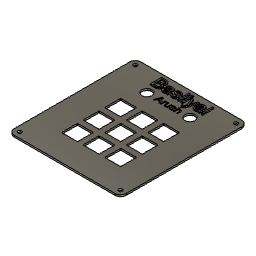
top part (Autodesk Fusion 360 design; units mm, degrees)
Autodesk Fusion 360 part; units mm, degrees
note: some values were not read from the file. Set by a fixed rule: which sketch regions a step uses.
(part 1 of 2)
sketch "plate-2025-07-12T03_53_15.257Z" plane through (0, 0, 0) normal (0, 0, 1) x (1, 0, 0)
  line L0 (3.025, -21.575) -> (16.025, -21.575)
  line L1 (3.025, -35.575) -> (16.025, -35.575)
  line L2 (2.525, -22.075) -> (2.525, -35.075)
  line L3 (16.525, -22.075) -> (16.525, -35.075)
  arc A0 (3.025, -21.575) -> (2.525, -22.075) centre (3.025, -22.075) ccw
  arc A1 (16.525, -22.075) -> (16.025, -21.575) centre (16.025, -22.075) ccw
  arc A2 (2.525, -35.075) -> (3.025, -35.575) centre (3.025, -35.075) ccw
  arc A3 (16.025, -35.575) -> (16.525, -35.075) centre (16.025, -35.075) ccw
  line L4 (22.075, -21.575) -> (35.075, -21.575)
  line L5 (22.075, -35.575) -> (35.075, -35.575)
  line L6 (21.575, -22.075) -> (21.575, -35.075)
  line L7 (35.575, -22.075) -> (35.575, -35.075)
  arc A4 (22.075, -21.575) -> (21.575, -22.075) centre (22.075, -22.075) ccw
  arc A5 (35.575, -22.075) -> (35.075, -21.575) centre (35.075, -22.075) ccw
  arc A6 (21.575, -35.075) -> (22.075, -35.575) centre (22.075, -35.075) ccw
  arc A7 (35.075, -35.575) -> (35.575, -35.075) centre (35.075, -35.075) ccw
  line L8 (41.125, -21.575) -> (54.125, -21.575)
  line L9 (41.125, -35.575) -> (54.125, -35.575)
  line L10 (40.625, -22.075) -> (40.625, -35.075)
  line L11 (54.625, -22.075) -> (54.625, -35.075)
  arc A8 (41.125, -21.575) -> (40.625, -22.075) centre (41.125, -22.075) ccw
  arc A9 (54.625, -22.075) -> (54.125, -21.575) centre (54.125, -22.075) ccw
  arc A10 (40.625, -35.075) -> (41.125, -35.575) centre (41.125, -35.075) ccw
  arc A11 (54.125, -35.575) -> (54.625, -35.075) centre (54.125, -35.075) ccw
  line L12 (3.025, -40.625) -> (16.025, -40.625)
  line L13 (3.025, -54.625) -> (16.025, -54.625)
  line L14 (2.525, -41.125) -> (2.525, -54.125)
  line L15 (16.525, -41.125) -> (16.525, -54.125)
  arc A12 (3.025, -40.625) -> (2.525, -41.125) centre (3.025, -41.125) ccw
  arc A13 (16.525, -41.125) -> (16.025, -40.625) centre (16.025, -41.125) ccw
  arc A14 (2.525, -54.125) -> (3.025, -54.625) centre (3.025, -54.125) ccw
  arc A15 (16.025, -54.625) -> (16.525, -54.125) centre (16.025, -54.125) ccw
  line L16 (22.075, -40.625) -> (35.075, -40.625)
  line L17 (22.075, -54.625) -> (35.075, -54.625)
  line L18 (21.575, -41.125) -> (21.575, -54.125)
  line L19 (35.575, -41.125) -> (35.575, -54.125)
  arc A16 (22.075, -40.625) -> (21.575, -41.125) centre (22.075, -41.125) ccw
  arc A17 (35.575, -41.125) -> (35.075, -40.625) centre (35.075, -41.125) ccw
  arc A18 (21.575, -54.125) -> (22.075, -54.625) centre (22.075, -54.125) ccw
  arc A19 (35.075, -54.625) -> (35.575, -54.125) centre (35.075, -54.125) ccw
  line L20 (41.125, -40.625) -> (54.125, -40.625)
  line L21 (41.125, -54.625) -> (54.125, -54.625)
  line L22 (40.625, -41.125) -> (40.625, -54.125)
  line L23 (54.625, -41.125) -> (54.625, -54.125)
  arc A20 (41.125, -40.625) -> (40.625, -41.125) centre (41.125, -41.125) ccw
  arc A21 (54.625, -41.125) -> (54.125, -40.625) centre (54.125, -41.125) ccw
  arc A22 (40.625, -54.125) -> (41.125, -54.625) centre (41.125, -54.125) ccw
  arc A23 (54.125, -54.625) -> (54.625, -54.125) centre (54.125, -54.125) ccw
  line L24 (3.025, -59.675) -> (16.025, -59.675)
  line L25 (3.025, -73.675) -> (16.025, -73.675)
  line L26 (2.525, -60.175) -> (2.525, -73.175)
  line L27 (16.525, -60.175) -> (16.525, -73.175)
  arc A24 (3.025, -59.675) -> (2.525, -60.175) centre (3.025, -60.175) ccw
  arc A25 (16.525, -60.175) -> (16.025, -59.675) centre (16.025, -60.175) ccw
  arc A26 (2.525, -73.175) -> (3.025, -73.675) centre (3.025, -73.175) ccw
  arc A27 (16.025, -73.675) -> (16.525, -73.175) centre (16.025, -73.175) ccw
  line L28 (22.075, -59.675) -> (35.075, -59.675)
  line L29 (22.075, -73.675) -> (35.075, -73.675)
  line L30 (21.575, -60.175) -> (21.575, -73.175)
  line L31 (35.575, -60.175) -> (35.575, -73.175)
  arc A28 (22.075, -59.675) -> (21.575, -60.175) centre (22.075, -60.175) ccw
  arc A29 (35.575, -60.175) -> (35.075, -59.675) centre (35.075, -60.175) ccw
  arc A30 (21.575, -73.175) -> (22.075, -73.675) centre (22.075, -73.175) ccw
  arc A31 (35.075, -73.675) -> (35.575, -73.175) centre (35.075, -73.175) ccw
  line L32 (41.125, -59.675) -> (54.125, -59.675)
  line L33 (41.125, -73.675) -> (54.125, -73.675)
  line L34 (40.625, -60.175) -> (40.625, -73.175)
  line L35 (54.625, -60.175) -> (54.625, -73.175)
  arc A32 (41.125, -59.675) -> (40.625, -60.175) centre (41.125, -60.175) ccw
  arc A33 (54.625, -60.175) -> (54.125, -59.675) centre (54.125, -60.175) ccw
  arc A34 (40.625, -73.175) -> (41.125, -73.675) centre (41.125, -73.175) ccw
  arc A35 (54.125, -73.675) -> (54.625, -73.175) centre (54.125, -73.175) ccw
sketch "Sketch2" plane through (0, 0, 0) normal (0, 0, 1) x (1, 0, 0)
  line L0 (-21.36, 15.31) -> (77.64, 15.31)
  line L1 (77.64, 15.31) -> (77.64, -96.69)
  line L2 (77.64, -96.69) -> (-21.36, -96.69)
  line L3 (-21.36, -96.69) -> (-21.36, 15.31)
  line L4 (54.625, -60.175) -> (54.625, -73.175)
  line L5 (41.125, -73.675) -> (54.125, -73.675)
  dimension "d1" = 99
  dimension "d2" = 112
  dimension "d3" = 23.015
  dimension "d4" = 23.015
  constraint horizontal L0
  constraint vertical L1
  constraint horizontal L2
  constraint vertical L3
  measures "d1" distance of L0.start L0.end
  measures "d2" distance of L0.start L2.end
  measures "d3" distance of L1 L4
  measures "d4" distance of L2 L5
sketch "Sketch3" plane through (0, 0, 0) normal (0, 0, 1) x (1, 0, 0)
  circle A0 centre (-16.36, 10.31) radius 1.7
  line L0 (-21.36, 15.31) -> (77.64, 15.31)
  line L1 (-21.36, -96.69) -> (-21.36, 15.31)
  circle A1 centre (72.64, 10.31) radius 1.7
  circle A2 centre (-16.36, -91.69) radius 1.7
  circle A3 centre (72.64, -91.69) radius 1.7
  dimension "d6" = 3.4
  dimension "d7" = 5
  dimension "d8" = 5
  measures "d6" diameter of A0
  measures "d7" distance of A0.centre L0
  measures "d8" distance of A0.centre L1
extrude "Extrude1" add sketch "Sketch2" along normal blind 1.5
extrude "Extrude2" cut sketch "plate-2025-07-12T03_53_15.257Z" sketch "Sketch3" along normal blind 1.5 of sketch 2
sketch "Sketch4" plane through (0, 0, 1.5) normal (0, 0, 1) x (-1, 0, 0)
  circle A0 centre (-72.64, 91.69) radius 1.7
  circle A1 centre (16.36, -10.31) radius 1.7
  line L0 (-41.125, 59.675) -> (-54.125, 59.675)
  arc A2 (-54.625, 60.175) -> (-54.125, 59.675) centre (-54.125, 60.175) ccw
  line L1 (-54.625, 60.175) -> (-54.625, 73.175)
  arc A3 (-54.125, 73.675) -> (-54.625, 73.175) centre (-54.125, 73.175) ccw
  line L2 (-54.125, 73.675) -> (-41.125, 73.675)
  arc A4 (-40.625, 73.175) -> (-41.125, 73.675) centre (-41.125, 73.175) ccw
  line L3 (-40.625, 73.175) -> (-40.625, 60.175)
  arc A5 (-41.125, 59.675) -> (-40.625, 60.175) centre (-41.125, 60.175) ccw
  line L4 (-3.025, 21.575) -> (-16.025, 21.575)
  arc A6 (-16.525, 22.075) -> (-16.025, 21.575) centre (-16.025, 22.075) ccw
  line L5 (-16.525, 22.075) -> (-16.525, 35.075)
  arc A7 (-16.025, 35.575) -> (-16.525, 35.075) centre (-16.025, 35.075) ccw
  line L6 (-16.025, 35.575) -> (-3.025, 35.575)
  arc A8 (-2.525, 35.075) -> (-3.025, 35.575) centre (-3.025, 35.075) ccw
  line L7 (-2.525, 35.075) -> (-2.525, 22.075)
  arc A9 (-3.025, 21.575) -> (-2.525, 22.075) centre (-3.025, 22.075) ccw
  line L8 (-22.075, 21.575) -> (-35.075, 21.575)
  arc A10 (-35.575, 22.075) -> (-35.075, 21.575) centre (-35.075, 22.075) ccw
  line L9 (-35.575, 22.075) -> (-35.575, 35.075)
  arc A11 (-35.075, 35.575) -> (-35.575, 35.075) centre (-35.075, 35.075) ccw
  line L10 (-35.075, 35.575) -> (-22.075, 35.575)
  arc A12 (-21.575, 35.075) -> (-22.075, 35.575) centre (-22.075, 35.075) ccw
  line L11 (-21.575, 35.075) -> (-21.575, 22.075)
  arc A13 (-22.075, 21.575) -> (-21.575, 22.075) centre (-22.075, 22.075) ccw
  line L12 (-41.125, 40.625) -> (-54.125, 40.625)
  arc A14 (-54.625, 41.125) -> (-54.125, 40.625) centre (-54.125, 41.125) ccw
  line L13 (-54.625, 41.125) -> (-54.625, 54.125)
  arc A15 (-54.125, 54.625) -> (-54.625, 54.125) centre (-54.125, 54.125) ccw
  line L14 (-54.125, 54.625) -> (-41.125, 54.625)
  arc A16 (-40.625, 54.125) -> (-41.125, 54.625) centre (-41.125, 54.125) ccw
  line L15 (-40.625, 54.125) -> (-40.625, 41.125)
  arc A17 (-41.125, 40.625) -> (-40.625, 41.125) centre (-41.125, 41.125) ccw
  line L16 (-22.075, 59.675) -> (-35.075, 59.675)
  arc A18 (-35.575, 60.175) -> (-35.075, 59.675) centre (-35.075, 60.175) ccw
  line L17 (-35.575, 60.175) -> (-35.575, 73.175)
  arc A19 (-35.075, 73.675) -> (-35.575, 73.175) centre (-35.075, 73.175) ccw
  line L18 (-35.075, 73.675) -> (-22.075, 73.675)
  arc A20 (-21.575, 73.175) -> (-22.075, 73.675) centre (-22.075, 73.175) ccw
  line L19 (-21.575, 73.175) -> (-21.575, 60.175)
  arc A21 (-22.075, 59.675) -> (-21.575, 60.175) centre (-22.075, 60.175) ccw
  line L20 (-3.025, 40.625) -> (-16.025, 40.625)
  arc A22 (-16.525, 41.125) -> (-16.025, 40.625) centre (-16.025, 41.125) ccw
  line L21 (-16.525, 41.125) -> (-16.525, 54.125)
  arc A23 (-16.025, 54.625) -> (-16.525, 54.125) centre (-16.025, 54.125) ccw
  line L22 (-16.025, 54.625) -> (-3.025, 54.625)
  arc A24 (-2.525, 54.125) -> (-3.025, 54.625) centre (-3.025, 54.125) ccw
  line L23 (-2.525, 54.125) -> (-2.525, 41.125)
  arc A25 (-3.025, 40.625) -> (-2.525, 41.125) centre (-3.025, 41.125) ccw
  line L24 (-41.125, 21.575) -> (-54.125, 21.575)
  arc A26 (-54.625, 22.075) -> (-54.125, 21.575) centre (-54.125, 22.075) ccw
  line L25 (-54.625, 22.075) -> (-54.625, 35.075)
  arc A27 (-54.125, 35.575) -> (-54.625, 35.075) centre (-54.125, 35.075) ccw
  line L26 (-54.125, 35.575) -> (-41.125, 35.575)
  arc A28 (-40.625, 35.075) -> (-41.125, 35.575) centre (-41.125, 35.075) ccw
  line L27 (-40.625, 35.075) -> (-40.625, 22.075)
  arc A29 (-41.125, 21.575) -> (-40.625, 22.075) centre (-41.125, 22.075) ccw
  line L28 (-22.075, 40.625) -> (-35.075, 40.625)
  arc A30 (-35.575, 41.125) -> (-35.075, 40.625) centre (-35.075, 41.125) ccw
  line L29 (-35.575, 41.125) -> (-35.575, 54.125)
  arc A31 (-35.075, 54.625) -> (-35.575, 54.125) centre (-35.075, 54.125) ccw
  line L30 (-35.075, 54.625) -> (-22.075, 54.625)
  arc A32 (-21.575, 54.125) -> (-22.075, 54.625) centre (-22.075, 54.125) ccw
  line L31 (-21.575, 54.125) -> (-21.575, 41.125)
  arc A33 (-22.075, 40.625) -> (-21.575, 41.125) centre (-22.075, 41.125) ccw
  line L32 (-3.025, 59.675) -> (-16.025, 59.675)
  arc A34 (-16.525, 60.175) -> (-16.025, 59.675) centre (-16.025, 60.175) ccw
  line L33 (-16.525, 60.175) -> (-16.525, 73.175)
  arc A35 (-16.025, 73.675) -> (-16.525, 73.175) centre (-16.025, 73.175) ccw
  line L34 (-16.025, 73.675) -> (-3.025, 73.675)
  arc A36 (-2.525, 73.175) -> (-3.025, 73.675) centre (-3.025, 73.175) ccw
  line L35 (-2.525, 73.175) -> (-2.525, 60.175)
  arc A37 (-3.025, 59.675) -> (-2.525, 60.175) centre (-3.025, 60.175) ccw
  circle A38 centre (16.36, 91.69) radius 1.7
  circle A39 centre (-72.64, -10.31) radius 1.7
  line L36 (21.36, 96.69) -> (-77.64, 96.69)
  line L37 (-77.64, 96.69) -> (-77.64, -15.31)
  line L38 (-77.64, -15.31) -> (21.36, -15.31)
  line L39 (21.36, -15.31) -> (21.36, 96.69)
  line L40 (-28.14, -15.31) -> (-28.14, 96.69)
  line L41 (-47.625, 28.575) -> (-28.14, 28.575)
  line L42 (-35.575, 47.625) -> (-28.14, 47.625)
  line L43 (-28.14, 47.625) -> (-28.14, 28.575)
  line L44 (-28.14, 28.575) -> (-28.14, 9.525)
  line L45 (-28.14, 9.525) -> (-47.625, 9.525)
  circle A40 centre (-47.625, 9.525) radius 4.25
  circle A41 centre (-8.655, 9.525) radius 4.25
  dimension "d13" = 19.05
  dimension "d14" = 8.5
  constraint midpoint L38 L40.start
  constraint midpoint L36 L40.end
  constraint coincident L40 L41.end
  constraint perpendicular L40 L41
  constraint midpoint L29 L42.start
  constraint coincident L40 L42.end
  constraint perpendicular L40 L42
  constraint perpendicular L41 L44
  constraint perpendicular L44 L45
  constraint coincident L45.end A40.centre
  constraint symmetric L40 A40 A41
  measures "d13" distance of L41.end L44.end
  measures "d14" diameter of A40
extrude "Extrude3" cut sketch "Sketch4" against normal blind 12 contours A40 | A41
fillet "Fillet1" radius 5 4 edges at (-21.36, -96.69, 0.75) (77.64, -96.69, 0.75) (77.64, 15.31, 0.75) (-21.36, 15.31, 0.75)
sketch "Sketch8" plane through (0, 0, 1.5) normal (0, 0, 1) x (-1, 0, 0)
  arc A0 (16.36, -15.31) -> (21.36, -10.31) centre (16.36, -10.31) ccw
  line L0 (21.36, -10.31) -> (21.36, 91.69)
  arc A1 (21.36, 91.69) -> (16.36, 96.69) centre (16.36, 91.69) ccw
  line L1 (16.36, 96.69) -> (-72.64, 96.69)
  arc A2 (-72.64, 96.69) -> (-77.64, 91.69) centre (-72.64, 91.69) ccw
  line L2 (-77.64, 91.69) -> (-77.64, -10.31)
  arc A3 (-77.64, -10.31) -> (-72.64, -15.31) centre (-72.64, -10.31) ccw
  line L3 (-72.64, -15.31) -> (16.36, -15.31)
  circle A4 centre (-72.64, -10.31) radius 1.7
  circle A5 centre (16.36, 91.69) radius 1.7
  line L4 (-3.025, 59.675) -> (-16.025, 59.675)
  arc A6 (-16.525, 60.175) -> (-16.025, 59.675) centre (-16.025, 60.175) ccw
  line L5 (-16.525, 60.175) -> (-16.525, 73.175)
  arc A7 (-16.025, 73.675) -> (-16.525, 73.175) centre (-16.025, 73.175) ccw
  line L6 (-16.025, 73.675) -> (-3.025, 73.675)
  arc A8 (-2.525, 73.175) -> (-3.025, 73.675) centre (-3.025, 73.175) ccw
  line L7 (-2.525, 73.175) -> (-2.525, 60.175)
  arc A9 (-3.025, 59.675) -> (-2.525, 60.175) centre (-3.025, 60.175) ccw
  line L8 (-22.075, 40.625) -> (-35.075, 40.625)
  arc A10 (-35.575, 41.125) -> (-35.075, 40.625) centre (-35.075, 41.125) ccw
  line L9 (-35.575, 41.125) -> (-35.575, 54.125)
  arc A11 (-35.075, 54.625) -> (-35.575, 54.125) centre (-35.075, 54.125) ccw
  line L10 (-35.075, 54.625) -> (-22.075, 54.625)
  arc A12 (-21.575, 54.125) -> (-22.075, 54.625) centre (-22.075, 54.125) ccw
  line L11 (-21.575, 54.125) -> (-21.575, 41.125)
  arc A13 (-22.075, 40.625) -> (-21.575, 41.125) centre (-22.075, 41.125) ccw
  line L12 (-41.125, 21.575) -> (-54.125, 21.575)
  arc A14 (-54.625, 22.075) -> (-54.125, 21.575) centre (-54.125, 22.075) ccw
  line L13 (-54.625, 22.075) -> (-54.625, 35.075)
  arc A15 (-54.125, 35.575) -> (-54.625, 35.075) centre (-54.125, 35.075) ccw
  line L14 (-54.125, 35.575) -> (-41.125, 35.575)
  arc A16 (-40.625, 35.075) -> (-41.125, 35.575) centre (-41.125, 35.075) ccw
  line L15 (-40.625, 35.075) -> (-40.625, 22.075)
  arc A17 (-41.125, 21.575) -> (-40.625, 22.075) centre (-41.125, 22.075) ccw
  line L16 (-3.025, 40.625) -> (-16.025, 40.625)
  arc A18 (-16.525, 41.125) -> (-16.025, 40.625) centre (-16.025, 41.125) ccw
  line L17 (-16.525, 41.125) -> (-16.525, 54.125)
  arc A19 (-16.025, 54.625) -> (-16.525, 54.125) centre (-16.025, 54.125) ccw
  line L18 (-16.025, 54.625) -> (-3.025, 54.625)
  arc A20 (-2.525, 54.125) -> (-3.025, 54.625) centre (-3.025, 54.125) ccw
  line L19 (-2.525, 54.125) -> (-2.525, 41.125)
  arc A21 (-3.025, 40.625) -> (-2.525, 41.125) centre (-3.025, 41.125) ccw
  line L20 (-22.075, 59.675) -> (-35.075, 59.675)
  arc A22 (-35.575, 60.175) -> (-35.075, 59.675) centre (-35.075, 60.175) ccw
  line L21 (-35.575, 60.175) -> (-35.575, 73.175)
  arc A23 (-35.075, 73.675) -> (-35.575, 73.175) centre (-35.075, 73.175) ccw
  line L22 (-35.075, 73.675) -> (-22.075, 73.675)
  arc A24 (-21.575, 73.175) -> (-22.075, 73.675) centre (-22.075, 73.175) ccw
  line L23 (-21.575, 73.175) -> (-21.575, 60.175)
  arc A25 (-22.075, 59.675) -> (-21.575, 60.175) centre (-22.075, 60.175) ccw
  line L24 (-41.125, 40.625) -> (-54.125, 40.625)
  arc A26 (-54.625, 41.125) -> (-54.125, 40.625) centre (-54.125, 41.125) ccw
  line L25 (-54.625, 41.125) -> (-54.625, 54.125)
  arc A27 (-54.125, 54.625) -> (-54.625, 54.125) centre (-54.125, 54.125) ccw
  line L26 (-54.125, 54.625) -> (-41.125, 54.625)
  arc A28 (-40.625, 54.125) -> (-41.125, 54.625) centre (-41.125, 54.125) ccw
  line L27 (-40.625, 54.125) -> (-40.625, 41.125)
  arc A29 (-41.125, 40.625) -> (-40.625, 41.125) centre (-41.125, 41.125) ccw
  line L28 (-22.075, 21.575) -> (-35.075, 21.575)
  arc A30 (-35.575, 22.075) -> (-35.075, 21.575) centre (-35.075, 22.075) ccw
  line L29 (-35.575, 22.075) -> (-35.575, 35.075)
  arc A31 (-35.075, 35.575) -> (-35.575, 35.075) centre (-35.075, 35.075) ccw
  line L30 (-35.075, 35.575) -> (-22.075, 35.575)
  arc A32 (-21.575, 35.075) -> (-22.075, 35.575) centre (-22.075, 35.075) ccw
  line L31 (-21.575, 35.075) -> (-21.575, 22.075)
  arc A33 (-22.075, 21.575) -> (-21.575, 22.075) centre (-22.075, 22.075) ccw
  line L32 (-3.025, 21.575) -> (-16.025, 21.575)
  arc A34 (-16.525, 22.075) -> (-16.025, 21.575) centre (-16.025, 22.075) ccw
  line L33 (-16.525, 22.075) -> (-16.525, 35.075)
  arc A35 (-16.025, 35.575) -> (-16.525, 35.075) centre (-16.025, 35.075) ccw
  line L34 (-16.025, 35.575) -> (-3.025, 35.575)
  arc A36 (-2.525, 35.075) -> (-3.025, 35.575) centre (-3.025, 35.075) ccw
  line L35 (-2.525, 35.075) -> (-2.525, 22.075)
  arc A37 (-3.025, 21.575) -> (-2.525, 22.075) centre (-3.025, 22.075) ccw
  line L36 (-41.125, 59.675) -> (-54.125, 59.675)
  arc A38 (-54.625, 60.175) -> (-54.125, 59.675) centre (-54.125, 60.175) ccw
  line L37 (-54.625, 60.175) -> (-54.625, 73.175)
  arc A39 (-54.125, 73.675) -> (-54.625, 73.175) centre (-54.125, 73.175) ccw
  line L38 (-54.125, 73.675) -> (-41.125, 73.675)
  arc A40 (-40.625, 73.175) -> (-41.125, 73.675) centre (-41.125, 73.175) ccw
  line L39 (-40.625, 73.175) -> (-40.625, 60.175)
  arc A41 (-41.125, 59.675) -> (-40.625, 60.175) centre (-41.125, 60.175) ccw
  circle A42 centre (16.36, -10.31) radius 1.7
  circle A43 centre (-72.64, 91.69) radius 1.7
  circle A44 centre (-8.655, 9.525) radius 4.25
  circle A45 centre (-47.625, 9.525) radius 4.25
sketch "Sketch9" plane through (0, 0, 1.5) normal (0, 0, 1) x (-1, 0, 0)
  arc A0 (16.36, -15.31) -> (21.36, -10.31) centre (16.36, -10.31) ccw
  line L0 (21.36, -10.31) -> (21.36, 91.69)
  arc A1 (21.36, 91.69) -> (16.36, 96.69) centre (16.36, 91.69) ccw
  line L1 (16.36, 96.69) -> (-72.64, 96.69)
  arc A2 (-72.64, 96.69) -> (-77.64, 91.69) centre (-72.64, 91.69) ccw
  line L2 (-77.64, 91.69) -> (-77.64, -10.31)
  arc A3 (-77.64, -10.31) -> (-72.64, -15.31) centre (-72.64, -10.31) ccw
  line L3 (-72.64, -15.31) -> (16.36, -15.31)
  circle A4 centre (-72.64, -10.31) radius 1.7
  circle A5 centre (16.36, 91.69) radius 1.7
  line L4 (-3.025, 59.675) -> (-16.025, 59.675)
  arc A6 (-16.525, 60.175) -> (-16.025, 59.675) centre (-16.025, 60.175) ccw
  line L5 (-16.525, 60.175) -> (-16.525, 73.175)
  arc A7 (-16.025, 73.675) -> (-16.525, 73.175) centre (-16.025, 73.175) ccw
  line L6 (-16.025, 73.675) -> (-3.025, 73.675)
  arc A8 (-2.525, 73.175) -> (-3.025, 73.675) centre (-3.025, 73.175) ccw
  line L7 (-2.525, 73.175) -> (-2.525, 60.175)
  arc A9 (-3.025, 59.675) -> (-2.525, 60.175) centre (-3.025, 60.175) ccw
  line L8 (-22.075, 40.625) -> (-35.075, 40.625)
  arc A10 (-35.575, 41.125) -> (-35.075, 40.625) centre (-35.075, 41.125) ccw
  line L9 (-35.575, 41.125) -> (-35.575, 54.125)
  arc A11 (-35.075, 54.625) -> (-35.575, 54.125) centre (-35.075, 54.125) ccw
  line L10 (-35.075, 54.625) -> (-22.075, 54.625)
  arc A12 (-21.575, 54.125) -> (-22.075, 54.625) centre (-22.075, 54.125) ccw
  line L11 (-21.575, 54.125) -> (-21.575, 41.125)
  arc A13 (-22.075, 40.625) -> (-21.575, 41.125) centre (-22.075, 41.125) ccw
  line L12 (-41.125, 21.575) -> (-54.125, 21.575)
  arc A14 (-54.625, 22.075) -> (-54.125, 21.575) centre (-54.125, 22.075) ccw
  line L13 (-54.625, 22.075) -> (-54.625, 35.075)
  arc A15 (-54.125, 35.575) -> (-54.625, 35.075) centre (-54.125, 35.075) ccw
  line L14 (-54.125, 35.575) -> (-41.125, 35.575)
  arc A16 (-40.625, 35.075) -> (-41.125, 35.575) centre (-41.125, 35.075) ccw
  line L15 (-40.625, 35.075) -> (-40.625, 22.075)
  arc A17 (-41.125, 21.575) -> (-40.625, 22.075) centre (-41.125, 22.075) ccw
  line L16 (-3.025, 40.625) -> (-16.025, 40.625)
  arc A18 (-16.525, 41.125) -> (-16.025, 40.625) centre (-16.025, 41.125) ccw
  line L17 (-16.525, 41.125) -> (-16.525, 54.125)
  arc A19 (-16.025, 54.625) -> (-16.525, 54.125) centre (-16.025, 54.125) ccw
  line L18 (-16.025, 54.625) -> (-3.025, 54.625)
  arc A20 (-2.525, 54.125) -> (-3.025, 54.625) centre (-3.025, 54.125) ccw
  line L19 (-2.525, 54.125) -> (-2.525, 41.125)
  arc A21 (-3.025, 40.625) -> (-2.525, 41.125) centre (-3.025, 41.125) ccw
  line L20 (-22.075, 59.675) -> (-35.075, 59.675)
  arc A22 (-35.575, 60.175) -> (-35.075, 59.675) centre (-35.075, 60.175) ccw
  line L21 (-35.575, 60.175) -> (-35.575, 73.175)
  arc A23 (-35.075, 73.675) -> (-35.575, 73.175) centre (-35.075, 73.175) ccw
  line L22 (-35.075, 73.675) -> (-22.075, 73.675)
  arc A24 (-21.575, 73.175) -> (-22.075, 73.675) centre (-22.075, 73.175) ccw
  line L23 (-21.575, 73.175) -> (-21.575, 60.175)
  arc A25 (-22.075, 59.675) -> (-21.575, 60.175) centre (-22.075, 60.175) ccw
  line L24 (-41.125, 40.625) -> (-54.125, 40.625)
  arc A26 (-54.625, 41.125) -> (-54.125, 40.625) centre (-54.125, 41.125) ccw
  line L25 (-54.625, 41.125) -> (-54.625, 54.125)
  arc A27 (-54.125, 54.625) -> (-54.625, 54.125) centre (-54.125, 54.125) ccw
  line L26 (-54.125, 54.625) -> (-41.125, 54.625)
  arc A28 (-40.625, 54.125) -> (-41.125, 54.625) centre (-41.125, 54.125) ccw
  line L27 (-40.625, 54.125) -> (-40.625, 41.125)
  arc A29 (-41.125, 40.625) -> (-40.625, 41.125) centre (-41.125, 41.125) ccw
  line L28 (-22.075, 21.575) -> (-35.075, 21.575)
  arc A30 (-35.575, 22.075) -> (-35.075, 21.575) centre (-35.075, 22.075) ccw
  line L29 (-35.575, 22.075) -> (-35.575, 35.075)
  arc A31 (-35.075, 35.575) -> (-35.575, 35.075) centre (-35.075, 35.075) ccw
  line L30 (-35.075, 35.575) -> (-22.075, 35.575)
  arc A32 (-21.575, 35.075) -> (-22.075, 35.575) centre (-22.075, 35.075) ccw
  line L31 (-21.575, 35.075) -> (-21.575, 22.075)
  arc A33 (-22.075, 21.575) -> (-21.575, 22.075) centre (-22.075, 22.075) ccw
  line L32 (-3.025, 21.575) -> (-16.025, 21.575)
  arc A34 (-16.525, 22.075) -> (-16.025, 21.575) centre (-16.025, 22.075) ccw
  line L33 (-16.525, 22.075) -> (-16.525, 35.075)
  arc A35 (-16.025, 35.575) -> (-16.525, 35.075) centre (-16.025, 35.075) ccw
  line L34 (-16.025, 35.575) -> (-3.025, 35.575)
  arc A36 (-2.525, 35.075) -> (-3.025, 35.575) centre (-3.025, 35.075) ccw
  line L35 (-2.525, 35.075) -> (-2.525, 22.075)
  arc A37 (-3.025, 21.575) -> (-2.525, 22.075) centre (-3.025, 22.075) ccw
  line L36 (-41.125, 59.675) -> (-54.125, 59.675)
  arc A38 (-54.625, 60.175) -> (-54.125, 59.675) centre (-54.125, 60.175) ccw
  line L37 (-54.625, 60.175) -> (-54.625, 73.175)
  arc A39 (-54.125, 73.675) -> (-54.625, 73.175) centre (-54.125, 73.175) ccw
  line L38 (-54.125, 73.675) -> (-41.125, 73.675)
  arc A40 (-40.625, 73.175) -> (-41.125, 73.675) centre (-41.125, 73.175) ccw
  line L39 (-40.625, 73.175) -> (-40.625, 60.175)
  arc A41 (-41.125, 59.675) -> (-40.625, 60.175) centre (-41.125, 60.175) ccw
  circle A42 centre (16.36, -10.31) radius 1.7
  circle A43 centre (-72.64, 91.69) radius 1.7
  circle A44 centre (-8.655, 9.525) radius 4.25
  circle A45 centre (-47.625, 9.525) radius 4.25
  line L40 (-0.3888, -0.9879) -> (-47.5126, -0.9879) construction
  line L41 (-47.5126, -0.9879) -> (-47.5126, -12.2261) construction
  line L42 (-47.5126, -12.2261) -> (-0.3888, -12.2261) construction
  line L43 (-0.3888, -12.2261) -> (-0.3888, -0.9879) construction
  dimension "d24" = 12
delete_face "DeleteFace1" 1 faces at (4.4261, -9.1018, 1)
delete_face "DeleteFace2" 1 faces at (43.3961, -9.1018, 1)
move_body "Move1" bodies 1 to x (1, 0, 0) y (0, 1, 0) z (0, 0, 1) at (0.6112, -1.4722, 0)
sketch "Sketch10" plane through (0, 0, 1.5) normal (0, 0, 1) x (-1, 0, 0)
  circle A0 centre (-73.2512, 93.1622) radius 1.7
  circle A1 centre (15.7488, -8.8378) radius 1.7
  line L0 (-41.7362, 61.1472) -> (-54.7362, 61.1472)
  arc A2 (-55.2362, 61.6472) -> (-54.7362, 61.1472) centre (-54.7362, 61.6472) ccw
  line L1 (-55.2362, 61.6472) -> (-55.2362, 74.6472)
  arc A3 (-54.7362, 75.1472) -> (-55.2362, 74.6472) centre (-54.7362, 74.6472) ccw
  line L2 (-54.7362, 75.1472) -> (-41.7362, 75.1472)
  arc A4 (-41.2362, 74.6472) -> (-41.7362, 75.1472) centre (-41.7362, 74.6472) ccw
  line L3 (-41.2362, 74.6472) -> (-41.2362, 61.6472)
  arc A5 (-41.7362, 61.1472) -> (-41.2362, 61.6472) centre (-41.7362, 61.6472) ccw
  line L4 (-3.6362, 23.0472) -> (-16.6362, 23.0472)
  arc A6 (-17.1362, 23.5472) -> (-16.6362, 23.0472) centre (-16.6362, 23.5472) ccw
  line L5 (-17.1362, 23.5472) -> (-17.1362, 36.5472)
  arc A7 (-16.6362, 37.0472) -> (-17.1362, 36.5472) centre (-16.6362, 36.5472) ccw
  line L6 (-16.6362, 37.0472) -> (-3.6362, 37.0472)
  arc A8 (-3.1362, 36.5472) -> (-3.6362, 37.0472) centre (-3.6362, 36.5472) ccw
  line L7 (-3.1362, 36.5472) -> (-3.1362, 23.5472)
  arc A9 (-3.6362, 23.0472) -> (-3.1362, 23.5472) centre (-3.6362, 23.5472) ccw
  line L8 (-22.6862, 23.0472) -> (-35.6862, 23.0472)
  arc A10 (-36.1862, 23.5472) -> (-35.6862, 23.0472) centre (-35.6862, 23.5472) ccw
  line L9 (-36.1862, 23.5472) -> (-36.1862, 36.5472)
  arc A11 (-35.6862, 37.0472) -> (-36.1862, 36.5472) centre (-35.6862, 36.5472) ccw
  line L10 (-35.6862, 37.0472) -> (-22.6862, 37.0472)
  arc A12 (-22.1862, 36.5472) -> (-22.6862, 37.0472) centre (-22.6862, 36.5472) ccw
  line L11 (-22.1862, 36.5472) -> (-22.1862, 23.5472)
  arc A13 (-22.6862, 23.0472) -> (-22.1862, 23.5472) centre (-22.6862, 23.5472) ccw
  line L12 (-41.7362, 42.0972) -> (-54.7362, 42.0972)
  arc A14 (-55.2362, 42.5972) -> (-54.7362, 42.0972) centre (-54.7362, 42.5972) ccw
  line L13 (-55.2362, 42.5972) -> (-55.2362, 55.5972)
  arc A15 (-54.7362, 56.0972) -> (-55.2362, 55.5972) centre (-54.7362, 55.5972) ccw
  line L14 (-54.7362, 56.0972) -> (-41.7362, 56.0972)
  arc A16 (-41.2362, 55.5972) -> (-41.7362, 56.0972) centre (-41.7362, 55.5972) ccw
  line L15 (-41.2362, 55.5972) -> (-41.2362, 42.5972)
  arc A17 (-41.7362, 42.0972) -> (-41.2362, 42.5972) centre (-41.7362, 42.5972) ccw
  line L16 (-22.6862, 61.1472) -> (-35.6862, 61.1472)
  arc A18 (-36.1862, 61.6472) -> (-35.6862, 61.1472) centre (-35.6862, 61.6472) ccw
  line L17 (-36.1862, 61.6472) -> (-36.1862, 74.6472)
  arc A19 (-35.6862, 75.1472) -> (-36.1862, 74.6472) centre (-35.6862, 74.6472) ccw
  line L18 (-35.6862, 75.1472) -> (-22.6862, 75.1472)
  arc A20 (-22.1862, 74.6472) -> (-22.6862, 75.1472) centre (-22.6862, 74.6472) ccw
  line L19 (-22.1862, 74.6472) -> (-22.1862, 61.6472)
  arc A21 (-22.6862, 61.1472) -> (-22.1862, 61.6472) centre (-22.6862, 61.6472) ccw
  line L20 (-3.6362, 42.0972) -> (-16.6362, 42.0972)
  arc A22 (-17.1362, 42.5972) -> (-16.6362, 42.0972) centre (-16.6362, 42.5972) ccw
  line L21 (-17.1362, 42.5972) -> (-17.1362, 55.5972)
  arc A23 (-16.6362, 56.0972) -> (-17.1362, 55.5972) centre (-16.6362, 55.5972) ccw
  line L22 (-16.6362, 56.0972) -> (-3.6362, 56.0972)
  arc A24 (-3.1362, 55.5972) -> (-3.6362, 56.0972) centre (-3.6362, 55.5972) ccw
  line L23 (-3.1362, 55.5972) -> (-3.1362, 42.5972)
  arc A25 (-3.6362, 42.0972) -> (-3.1362, 42.5972) centre (-3.6362, 42.5972) ccw
  line L24 (-41.7362, 23.0472) -> (-54.7362, 23.0472)
  arc A26 (-55.2362, 23.5472) -> (-54.7362, 23.0472) centre (-54.7362, 23.5472) ccw
  line L25 (-55.2362, 23.5472) -> (-55.2362, 36.5472)
  arc A27 (-54.7362, 37.0472) -> (-55.2362, 36.5472) centre (-54.7362, 36.5472) ccw
  line L26 (-54.7362, 37.0472) -> (-41.7362, 37.0472)
  arc A28 (-41.2362, 36.5472) -> (-41.7362, 37.0472) centre (-41.7362, 36.5472) ccw
  line L27 (-41.2362, 36.5472) -> (-41.2362, 23.5472)
  arc A29 (-41.7362, 23.0472) -> (-41.2362, 23.5472) centre (-41.7362, 23.5472) ccw
  line L28 (-22.6862, 42.0972) -> (-35.6862, 42.0972)
  arc A30 (-36.1862, 42.5972) -> (-35.6862, 42.0972) centre (-35.6862, 42.5972) ccw
  line L29 (-36.1862, 42.5972) -> (-36.1862, 55.5972)
  arc A31 (-35.6862, 56.0972) -> (-36.1862, 55.5972) centre (-35.6862, 55.5972) ccw
  line L30 (-35.6862, 56.0972) -> (-22.6862, 56.0972)
  arc A32 (-22.1862, 55.5972) -> (-22.6862, 56.0972) centre (-22.6862, 55.5972) ccw
  line L31 (-22.1862, 55.5972) -> (-22.1862, 42.5972)
  arc A33 (-22.6862, 42.0972) -> (-22.1862, 42.5972) centre (-22.6862, 42.5972) ccw
  line L32 (-3.6362, 61.1472) -> (-16.6362, 61.1472)
  arc A34 (-17.1362, 61.6472) -> (-16.6362, 61.1472) centre (-16.6362, 61.6472) ccw
  line L33 (-17.1362, 61.6472) -> (-17.1362, 74.6472)
  arc A35 (-16.6362, 75.1472) -> (-17.1362, 74.6472) centre (-16.6362, 74.6472) ccw
  line L34 (-16.6362, 75.1472) -> (-3.6362, 75.1472)
  arc A36 (-3.1362, 74.6472) -> (-3.6362, 75.1472) centre (-3.6362, 74.6472) ccw
  line L35 (-3.1362, 74.6472) -> (-3.1362, 61.6472)
  arc A37 (-3.6362, 61.1472) -> (-3.1362, 61.6472) centre (-3.6362, 61.6472) ccw
  circle A38 centre (15.7488, 93.1622) radius 1.7
  circle A39 centre (-73.2512, -8.8378) radius 1.7
  arc A40 (15.7488, -13.8378) -> (20.7488, -8.8378) centre (15.7488, -8.8378) ccw
  line L36 (20.7488, -8.8378) -> (20.7488, 93.1622)
  arc A41 (20.7488, 93.1622) -> (15.7488, 98.1622) centre (15.7488, 93.1622) ccw
  line L37 (15.7488, 98.1622) -> (-73.2512, 98.1622)
  arc A42 (-73.2512, 98.1622) -> (-78.2512, 93.1622) centre (-73.2512, 93.1622) ccw
  line L38 (-78.2512, 93.1622) -> (-78.2512, -8.8378)
  arc A43 (-78.2512, -8.8378) -> (-73.2512, -13.8378) centre (-73.2512, -8.8378) ccw
  line L39 (-73.2512, -13.8378) -> (15.7488, -13.8378)
  line L40 (-29.1862, 49.0972) -> (-28.7512, -13.8378)
  circle A44 centre (-10.3772, 7.104) radius 4.5
  circle A45 centre (-47.4129, 6.848) radius 4.5
  dimension "d27" = 9
  constraint midpoint L39 L40.end
  constraint symmetric L40 A44 A45
  measures "d27" diameter of A44
extrude "Extrude7" cut sketch "Sketch10" against normal blind 5 contours A44 | A45
delete_face "DeleteFace3" 1 faces at (42.9353, -6.4, 1)
sketch "Sketch11" plane through (0, 0, 1.5) normal (0, 0, 1) x (-1, 0, 0)
  circle A0 centre (-10.3772, 7.104) radius 4.5
  circle A1 centre (-73.2512, 93.1622) radius 1.7
  circle A2 centre (15.7488, -8.8378) radius 1.7
  line L0 (-41.7362, 61.1472) -> (-54.7362, 61.1472)
  arc A3 (-55.2362, 61.6472) -> (-54.7362, 61.1472) centre (-54.7362, 61.6472) ccw
  line L1 (-55.2362, 61.6472) -> (-55.2362, 74.6472)
  arc A4 (-54.7362, 75.1472) -> (-55.2362, 74.6472) centre (-54.7362, 74.6472) ccw
  line L2 (-54.7362, 75.1472) -> (-41.7362, 75.1472)
  arc A5 (-41.2362, 74.6472) -> (-41.7362, 75.1472) centre (-41.7362, 74.6472) ccw
  line L3 (-41.2362, 74.6472) -> (-41.2362, 61.6472)
  arc A6 (-41.7362, 61.1472) -> (-41.2362, 61.6472) centre (-41.7362, 61.6472) ccw
  line L4 (-3.6362, 23.0472) -> (-16.6362, 23.0472)
  arc A7 (-17.1362, 23.5472) -> (-16.6362, 23.0472) centre (-16.6362, 23.5472) ccw
  line L5 (-17.1362, 23.5472) -> (-17.1362, 36.5472)
  arc A8 (-16.6362, 37.0472) -> (-17.1362, 36.5472) centre (-16.6362, 36.5472) ccw
  line L6 (-16.6362, 37.0472) -> (-3.6362, 37.0472)
  arc A9 (-3.1362, 36.5472) -> (-3.6362, 37.0472) centre (-3.6362, 36.5472) ccw
  line L7 (-3.1362, 36.5472) -> (-3.1362, 23.5472)
  arc A10 (-3.6362, 23.0472) -> (-3.1362, 23.5472) centre (-3.6362, 23.5472) ccw
  line L8 (-22.6862, 23.0472) -> (-35.6862, 23.0472)
  arc A11 (-36.1862, 23.5472) -> (-35.6862, 23.0472) centre (-35.6862, 23.5472) ccw
  line L9 (-36.1862, 23.5472) -> (-36.1862, 36.5472)
  arc A12 (-35.6862, 37.0472) -> (-36.1862, 36.5472) centre (-35.6862, 36.5472) ccw
  line L10 (-35.6862, 37.0472) -> (-22.6862, 37.0472)
  arc A13 (-22.1862, 36.5472) -> (-22.6862, 37.0472) centre (-22.6862, 36.5472) ccw
  line L11 (-22.1862, 36.5472) -> (-22.1862, 23.5472)
  arc A14 (-22.6862, 23.0472) -> (-22.1862, 23.5472) centre (-22.6862, 23.5472) ccw
  line L12 (-41.7362, 42.0972) -> (-54.7362, 42.0972)
  arc A15 (-55.2362, 42.5972) -> (-54.7362, 42.0972) centre (-54.7362, 42.5972) ccw
  line L13 (-55.2362, 42.5972) -> (-55.2362, 55.5972)
  arc A16 (-54.7362, 56.0972) -> (-55.2362, 55.5972) centre (-54.7362, 55.5972) ccw
  line L14 (-54.7362, 56.0972) -> (-41.7362, 56.0972)
  arc A17 (-41.2362, 55.5972) -> (-41.7362, 56.0972) centre (-41.7362, 55.5972) ccw
  line L15 (-41.2362, 55.5972) -> (-41.2362, 42.5972)
  arc A18 (-41.7362, 42.0972) -> (-41.2362, 42.5972) centre (-41.7362, 42.5972) ccw
  line L16 (-22.6862, 61.1472) -> (-35.6862, 61.1472)
  arc A19 (-36.1862, 61.6472) -> (-35.6862, 61.1472) centre (-35.6862, 61.6472) ccw
  line L17 (-36.1862, 61.6472) -> (-36.1862, 74.6472)
  arc A20 (-35.6862, 75.1472) -> (-36.1862, 74.6472) centre (-35.6862, 74.6472) ccw
  line L18 (-35.6862, 75.1472) -> (-22.6862, 75.1472)
  arc A21 (-22.1862, 74.6472) -> (-22.6862, 75.1472) centre (-22.6862, 74.6472) ccw
  line L19 (-22.1862, 74.6472) -> (-22.1862, 61.6472)
  arc A22 (-22.6862, 61.1472) -> (-22.1862, 61.6472) centre (-22.6862, 61.6472) ccw
  line L20 (-3.6362, 42.0972) -> (-16.6362, 42.0972)
  arc A23 (-17.1362, 42.5972) -> (-16.6362, 42.0972) centre (-16.6362, 42.5972) ccw
  line L21 (-17.1362, 42.5972) -> (-17.1362, 55.5972)
  arc A24 (-16.6362, 56.0972) -> (-17.1362, 55.5972) centre (-16.6362, 55.5972) ccw
  line L22 (-16.6362, 56.0972) -> (-3.6362, 56.0972)
  arc A25 (-3.1362, 55.5972) -> (-3.6362, 56.0972) centre (-3.6362, 55.5972) ccw
  line L23 (-3.1362, 55.5972) -> (-3.1362, 42.5972)
  arc A26 (-3.6362, 42.0972) -> (-3.1362, 42.5972) centre (-3.6362, 42.5972) ccw
  line L24 (-41.7362, 23.0472) -> (-54.7362, 23.0472)
  arc A27 (-55.2362, 23.5472) -> (-54.7362, 23.0472) centre (-54.7362, 23.5472) ccw
  line L25 (-55.2362, 23.5472) -> (-55.2362, 36.5472)
  arc A28 (-54.7362, 37.0472) -> (-55.2362, 36.5472) centre (-54.7362, 36.5472) ccw
  line L26 (-54.7362, 37.0472) -> (-41.7362, 37.0472)
  arc A29 (-41.2362, 36.5472) -> (-41.7362, 37.0472) centre (-41.7362, 36.5472) ccw
  line L27 (-41.2362, 36.5472) -> (-41.2362, 23.5472)
  arc A30 (-41.7362, 23.0472) -> (-41.2362, 23.5472) centre (-41.7362, 23.5472) ccw
  line L28 (-22.6862, 42.0972) -> (-35.6862, 42.0972)
  arc A31 (-36.1862, 42.5972) -> (-35.6862, 42.0972) centre (-35.6862, 42.5972) ccw
  line L29 (-36.1862, 42.5972) -> (-36.1862, 55.5972)
  arc A32 (-35.6862, 56.0972) -> (-36.1862, 55.5972) centre (-35.6862, 55.5972) ccw
  line L30 (-35.6862, 56.0972) -> (-22.6862, 56.0972)
  arc A33 (-22.1862, 55.5972) -> (-22.6862, 56.0972) centre (-22.6862, 55.5972) ccw
  line L31 (-22.1862, 55.5972) -> (-22.1862, 42.5972)
  arc A34 (-22.6862, 42.0972) -> (-22.1862, 42.5972) centre (-22.6862, 42.5972) ccw
  line L32 (-3.6362, 61.1472) -> (-16.6362, 61.1472)
  arc A35 (-17.1362, 61.6472) -> (-16.6362, 61.1472) centre (-16.6362, 61.6472) ccw
  line L33 (-17.1362, 61.6472) -> (-17.1362, 74.6472)
  arc A36 (-16.6362, 75.1472) -> (-17.1362, 74.6472) centre (-16.6362, 74.6472) ccw
  line L34 (-16.6362, 75.1472) -> (-3.6362, 75.1472)
  arc A37 (-3.1362, 74.6472) -> (-3.6362, 75.1472) centre (-3.6362, 74.6472) ccw
  line L35 (-3.1362, 74.6472) -> (-3.1362, 61.6472)
  arc A38 (-3.6362, 61.1472) -> (-3.1362, 61.6472) centre (-3.6362, 61.6472) ccw
  circle A39 centre (15.7488, 93.1622) radius 1.7
  circle A40 centre (-73.2512, -8.8378) radius 1.7
  arc A41 (15.7488, -13.8378) -> (20.7488, -8.8378) centre (15.7488, -8.8378) ccw
  line L36 (20.7488, -8.8378) -> (20.7488, 93.1622)
  arc A42 (20.7488, 93.1622) -> (15.7488, 98.1622) centre (15.7488, 93.1622) ccw
  line L37 (15.7488, 98.1622) -> (-73.2512, 98.1622)
  arc A43 (-73.2512, 98.1622) -> (-78.2512, 93.1622) centre (-73.2512, 93.1622) ccw
  line L38 (-78.2512, 93.1622) -> (-78.2512, -8.8378)
  arc A44 (-78.2512, -8.8378) -> (-73.2512, -13.8378) centre (-73.2512, -8.8378) ccw
  line L39 (-73.2512, -13.8378) -> (15.7488, -13.8378)
  line L40 (-10.3772, 7.104) -> (-78.2512, 7.104)
  line L41 (-48.3914, 3.588) -> (-48.3914, 10.5864)
  circle A45 centre (-48.3914, 7.0872) radius 4.75
  dimension "d30" = 9.5
  constraint coincident A0.centre L40.start
  constraint coincident L38 L40.end
  constraint perpendicular L38 L40
  constraint perpendicular L40 L41
  constraint midpoint L41 A45.centre
  measures "d30" diameter of A45
extrude "Extrude8" cut sketch "Sketch11" against normal blind 3 contours L40 A45 | L40 A45
sketch "Sketch12" plane through (0, 0, 1.5) normal (0, 0, 1) x (-1, 0, 0)
  circle A0 centre (-48.3914, 7.0872) radius 4.75
  circle A1 centre (-10.3772, 7.104) radius 4.5
  circle A2 centre (-73.2512, 93.1622) radius 1.7
  circle A3 centre (15.7488, -8.8378) radius 1.7
  line L0 (-41.7362, 61.1472) -> (-54.7362, 61.1472)
  arc A4 (-55.2362, 61.6472) -> (-54.7362, 61.1472) centre (-54.7362, 61.6472) ccw
  line L1 (-55.2362, 61.6472) -> (-55.2362, 74.6472)
  arc A5 (-54.7362, 75.1472) -> (-55.2362, 74.6472) centre (-54.7362, 74.6472) ccw
  line L2 (-54.7362, 75.1472) -> (-41.7362, 75.1472)
  arc A6 (-41.2362, 74.6472) -> (-41.7362, 75.1472) centre (-41.7362, 74.6472) ccw
  line L3 (-41.2362, 74.6472) -> (-41.2362, 61.6472)
  arc A7 (-41.7362, 61.1472) -> (-41.2362, 61.6472) centre (-41.7362, 61.6472) ccw
  line L4 (-3.6362, 23.0472) -> (-16.6362, 23.0472)
  arc A8 (-17.1362, 23.5472) -> (-16.6362, 23.0472) centre (-16.6362, 23.5472) ccw
  line L5 (-17.1362, 23.5472) -> (-17.1362, 36.5472)
  arc A9 (-16.6362, 37.0472) -> (-17.1362, 36.5472) centre (-16.6362, 36.5472) ccw
  line L6 (-16.6362, 37.0472) -> (-3.6362, 37.0472)
  arc A10 (-3.1362, 36.5472) -> (-3.6362, 37.0472) centre (-3.6362, 36.5472) ccw
  line L7 (-3.1362, 36.5472) -> (-3.1362, 23.5472)
  arc A11 (-3.6362, 23.0472) -> (-3.1362, 23.5472) centre (-3.6362, 23.5472) ccw
  line L8 (-22.6862, 23.0472) -> (-35.6862, 23.0472)
  arc A12 (-36.1862, 23.5472) -> (-35.6862, 23.0472) centre (-35.6862, 23.5472) ccw
  line L9 (-36.1862, 23.5472) -> (-36.1862, 36.5472)
  arc A13 (-35.6862, 37.0472) -> (-36.1862, 36.5472) centre (-35.6862, 36.5472) ccw
  line L10 (-35.6862, 37.0472) -> (-22.6862, 37.0472)
  arc A14 (-22.1862, 36.5472) -> (-22.6862, 37.0472) centre (-22.6862, 36.5472) ccw
  line L11 (-22.1862, 36.5472) -> (-22.1862, 23.5472)
  arc A15 (-22.6862, 23.0472) -> (-22.1862, 23.5472) centre (-22.6862, 23.5472) ccw
  line L12 (-41.7362, 42.0972) -> (-54.7362, 42.0972)
  arc A16 (-55.2362, 42.5972) -> (-54.7362, 42.0972) centre (-54.7362, 42.5972) ccw
  line L13 (-55.2362, 42.5972) -> (-55.2362, 55.5972)
  arc A17 (-54.7362, 56.0972) -> (-55.2362, 55.5972) centre (-54.7362, 55.5972) ccw
  line L14 (-54.7362, 56.0972) -> (-41.7362, 56.0972)
  arc A18 (-41.2362, 55.5972) -> (-41.7362, 56.0972) centre (-41.7362, 55.5972) ccw
  line L15 (-41.2362, 55.5972) -> (-41.2362, 42.5972)
  arc A19 (-41.7362, 42.0972) -> (-41.2362, 42.5972) centre (-41.7362, 42.5972) ccw
  line L16 (-22.6862, 61.1472) -> (-35.6862, 61.1472)
  arc A20 (-36.1862, 61.6472) -> (-35.6862, 61.1472) centre (-35.6862, 61.6472) ccw
  line L17 (-36.1862, 61.6472) -> (-36.1862, 74.6472)
  arc A21 (-35.6862, 75.1472) -> (-36.1862, 74.6472) centre (-35.6862, 74.6472) ccw
  line L18 (-35.6862, 75.1472) -> (-22.6862, 75.1472)
  arc A22 (-22.1862, 74.6472) -> (-22.6862, 75.1472) centre (-22.6862, 74.6472) ccw
  line L19 (-22.1862, 74.6472) -> (-22.1862, 61.6472)
  arc A23 (-22.6862, 61.1472) -> (-22.1862, 61.6472) centre (-22.6862, 61.6472) ccw
  line L20 (-3.6362, 42.0972) -> (-16.6362, 42.0972)
  arc A24 (-17.1362, 42.5972) -> (-16.6362, 42.0972) centre (-16.6362, 42.5972) ccw
  line L21 (-17.1362, 42.5972) -> (-17.1362, 55.5972)
  arc A25 (-16.6362, 56.0972) -> (-17.1362, 55.5972) centre (-16.6362, 55.5972) ccw
  line L22 (-16.6362, 56.0972) -> (-3.6362, 56.0972)
  arc A26 (-3.1362, 55.5972) -> (-3.6362, 56.0972) centre (-3.6362, 55.5972) ccw
  line L23 (-3.1362, 55.5972) -> (-3.1362, 42.5972)
  arc A27 (-3.6362, 42.0972) -> (-3.1362, 42.5972) centre (-3.6362, 42.5972) ccw
  line L24 (-41.7362, 23.0472) -> (-54.7362, 23.0472)
  arc A28 (-55.2362, 23.5472) -> (-54.7362, 23.0472) centre (-54.7362, 23.5472) ccw
  line L25 (-55.2362, 23.5472) -> (-55.2362, 36.5472)
  arc A29 (-54.7362, 37.0472) -> (-55.2362, 36.5472) centre (-54.7362, 36.5472) ccw
  line L26 (-54.7362, 37.0472) -> (-41.7362, 37.0472)
  arc A30 (-41.2362, 36.5472) -> (-41.7362, 37.0472) centre (-41.7362, 36.5472) ccw
  line L27 (-41.2362, 36.5472) -> (-41.2362, 23.5472)
  arc A31 (-41.7362, 23.0472) -> (-41.2362, 23.5472) centre (-41.7362, 23.5472) ccw
  line L28 (-22.6862, 42.0972) -> (-35.6862, 42.0972)
  arc A32 (-36.1862, 42.5972) -> (-35.6862, 42.0972) centre (-35.6862, 42.5972) ccw
  line L29 (-36.1862, 42.5972) -> (-36.1862, 55.5972)
  arc A33 (-35.6862, 56.0972) -> (-36.1862, 55.5972) centre (-35.6862, 55.5972) ccw
  line L30 (-35.6862, 56.0972) -> (-22.6862, 56.0972)
  arc A34 (-22.1862, 55.5972) -> (-22.6862, 56.0972) centre (-22.6862, 55.5972) ccw
  line L31 (-22.1862, 55.5972) -> (-22.1862, 42.5972)
  arc A35 (-22.6862, 42.0972) -> (-22.1862, 42.5972) centre (-22.6862, 42.5972) ccw
  line L32 (-3.6362, 61.1472) -> (-16.6362, 61.1472)
  arc A36 (-17.1362, 61.6472) -> (-16.6362, 61.1472) centre (-16.6362, 61.6472) ccw
  line L33 (-17.1362, 61.6472) -> (-17.1362, 74.6472)
  arc A37 (-16.6362, 75.1472) -> (-17.1362, 74.6472) centre (-16.6362, 74.6472) ccw
  line L34 (-16.6362, 75.1472) -> (-3.6362, 75.1472)
  arc A38 (-3.1362, 74.6472) -> (-3.6362, 75.1472) centre (-3.6362, 74.6472) ccw
  line L35 (-3.1362, 74.6472) -> (-3.1362, 61.6472)
  arc A39 (-3.6362, 61.1472) -> (-3.1362, 61.6472) centre (-3.6362, 61.6472) ccw
  circle A40 centre (15.7488, 93.1622) radius 1.7
  circle A41 centre (-73.2512, -8.8378) radius 1.7
  arc A42 (15.7488, -13.8378) -> (20.7488, -8.8378) centre (15.7488, -8.8378) ccw
  line L36 (20.7488, -8.8378) -> (20.7488, 93.1622)
  arc A43 (20.7488, 93.1622) -> (15.7488, 98.1622) centre (15.7488, 93.1622) ccw
  line L37 (15.7488, 98.1622) -> (-73.2512, 98.1622)
  arc A44 (-73.2512, 98.1622) -> (-78.2512, 93.1622) centre (-73.2512, 93.1622) ccw
  line L38 (-78.2512, 93.1622) -> (-78.2512, -8.8378)
  arc A45 (-78.2512, -8.8378) -> (-73.2512, -13.8378) centre (-73.2512, -8.8378) ccw
  line L39 (-73.2512, -13.8378) -> (15.7488, -13.8378)
  line L40 (-18.4165, 10.5379) -> (-36.758, 10.5379) construction
  line L41 (-36.758, 10.5379) -> (-36.758, 3.6351) construction
  line L42 (-36.758, 3.6351) -> (-18.4165, 3.6351) construction
  line L43 (-18.4165, 3.6351) -> (-18.4165, 10.5379) construction
  line L44 (-6.1342, -0.8273) -> (-55.6476, -0.8273) construction
  line L45 (-55.6476, -0.8273) -> (-55.6476, -10.2087) construction
  line L46 (-55.6476, -10.2087) -> (-6.1342, -10.2087) construction
  line L47 (-6.1342, -10.2087) -> (-6.1342, -0.8273) construction
  dimension "d33" = 6
  dimension "d34" = 10
  text T0 "Arush" font "Arial" height 6 align left top in box 18.3416 x 6.9027 at (-18.4165, 10.5379) x (-1, 0) y (0, -1) spacing 1
  text T1 "Basliyal" font "Arial" height 10 align left top in box 49.5134 x 9.3815 at (-6.1342, -0.8273) x (-1, 0) y (0, -1) spacing 1
extrude "Extrude9" cut sketch "Sketch12" against normal blind 0.1 text T0
sketch "Sketch13" plane through (0, 0, 1.5) normal (0, 0, 1) x (1, 0, 0)
extrude "Extrude10" add sketch "Sketch12" along normal blind 1 text T1